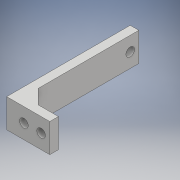
# Autodesk Inventor part: equerre-bras
Saved by Autodesk Inventor 2017 (Build 210142000, 142)
## iProperties
Created: 2018-04-01
Part Number: equerre-bras
Material: Generic
Document SubType Name: Modeling
Designer: franc
Density: 1 g/cm^3
Appearance: Default
Author: franc
Autodesk Inventor part; units mm, degrees
ref_plane "YZ Plane" through (0, 0, 0) normal (1, 0, 0) x (0, 1, 0)
ref_plane "XZ Plane" through (0, 0, 0) normal (0, 1, 0) x (-1, 0, 0)
ref_plane "XY Plane" through (0, 0, 0) normal (0, 0, 1) x (1, 0, 0)
sketch "Esquisse1" plane through (0, 0, 0) normal (0, 1, 0) x (-1, 0, 0)
  line L0 (2.8537, 2.5756) -> (-12.1463, 2.5756)
  line L1 (-12.1463, 2.5756) -> (-12.1463, -7.4244)
  line L2 (-12.1463, -7.4244) -> (2.8537, -7.4244)
  line L3 (2.8537, -7.4244) -> (2.8537, 2.5756)
  point P0 (0, 0)
  dimension "d0" = 10
  dimension "d1" = 15
  constraints: 8 end point, 2 parallel, 1 horizontal, 1 perpendicular
  measures "d0" distance of L2.end L0.start
  measures "d1" distance of L0.start L0.end
extrude "Extrusion1" add sketch "Esquisse1" along normal blind 3
sketch "Esquisse2" plane through (0, 3, 0) normal (0, 1, 0) x (1, 0, 0)
  line L0 (-2.8537, 7.4244) -> (-2.8537, -2.5756) projected
  line L1 (12.1463, 7.4244) -> (-2.8537, 7.4244) projected
  line L2 (-2.8537, -2.5756) -> (0.1463, -2.5756)
  line L3 (0.1463, -2.5756) -> (0.1463, 7.4244)
  line L4 (0.1463, 7.4244) -> (-2.8537, 7.4244)
  line L5 (-2.8537, 7.4244) -> (-2.8537, -2.5756)
  point P0 (0, 0)
  dimension "d4" = 3
  constraints: 8 end point, 2 parallel, 1 horizontal, 1 perpendicular, 1 point on line
  measures "d4" distance of L0.end L2.end
extrude "Extrusion2" add sketch "Esquisse2" along normal blind 40
sketch "Esquisse3" plane through (0, 3, 0) normal (0, 1, 0) x (1, 0, 0)
  circle A0 centre (3.1463, 2.4244) radius 1.5
  circle A1 centre (9.1463, 2.4244) radius 1.5
  line L0 (12.1463, -2.5756) -> (12.1463, 7.4244) projected
  line L1 (0.1463, -2.5756) -> (12.1463, -2.5756) projected
  line L2 (0.1463, -2.5756) -> (0.1463, 7.4244) projected
  point P0 (0, 0)
  dimension "d7" = 3
  dimension "d8" = 3
  dimension "d9" = 3
  dimension "d10" = 5
  dimension "d11" = 5
  dimension "d12" = 3
  constraints: 2 centre point
  measures "d7" diameter of A0
  measures "d8" diameter of A1
  measures "d9" distance from line of L0 A1.centre
  measures "d10" distance from line of L1 A1.centre
  measures "d11" distance from line of L1 A0.centre
  measures "d12" distance from line of L2 A0.centre
extrude "Extrusion3" cut sketch "Esquisse3" against normal through all
sketch "Esquisse4" plane through (0, 3, 0) normal (0, 1, 0) x (1, 0, 0)
  line L0 (0.1463, -2.5756) -> (12.1463, -2.5756) projected
  line L1 (0.1463, -2.5756) -> (5.1463, -2.5756)
  line L2 (5.1463, -2.5756) -> (5.1463, -1.5756)
  line L3 (5.1463, -1.5756) -> (0.1463, -1.5756)
  line L4 (0.1463, -1.5756) -> (0.1463, -2.5756)
  line L5 (12.1463, 7.4244) -> (0.1463, 7.4244) projected
  line L6 (0.1463, 7.4244) -> (5.1463, 7.4244)
  line L7 (5.1463, 7.4244) -> (5.1463, 6.4244)
  line L8 (5.1463, 6.4244) -> (0.1463, 6.4244)
  line L9 (0.1463, 6.4244) -> (0.1463, 7.4244)
  point P0 (0, 0)
  dimension "d15" = 1
  dimension "d16" = 1
  dimension "d17" = 5
  constraints: 16 end point, 4 parallel, 2 horizontal, 2 perpendicular, 1 point on line
  measures "d15" distance of L1.end L2.end
  measures "d16" distance of L6.end L7.end
  measures "d17" distance of L2.end L3.end
extrude "Extrusion4" add sketch "Esquisse4" along normal blind 5
chamfer "Chanfrein1" distance 5 angle 45 1 edges at (5.1463, 8, 2.0756)
chamfer "Chanfrein2" distance 5 angle 45 1 edges at (5.1463, 8, -6.9244)
sketch "Esquisse5" plane through (0.1463, 43, 2.5756) normal (1, 0, 0) x (0, 0, -1)
  circle A0 centre (5, -3) radius 1.5
  line L0 (0, -35) -> (0, 0) projected
  line L1 (0, 0) -> (10, 0) projected
  point P0 (2.5756, -43)
  dimension "d26" = 3
  dimension "d27" = 5
  dimension "d28" = 3
  constraints: 1 centre point
  measures "d26" diameter of A0
  measures "d27" distance from line of L0 A0.centre
  measures "d28" distance from line of A0.centre L1
extrude "Extrusion5" cut sketch "Esquisse5" against normal through all
